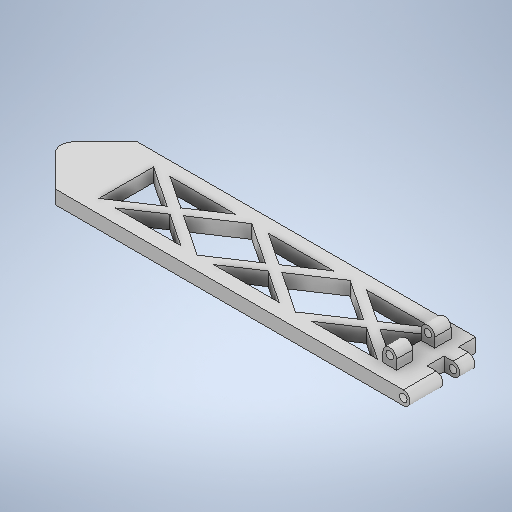
# Autodesk Inventor part: scrambler_spider_beam
Saved by Autodesk Inventor 2025.2 (Build 292293000, 293)
## iProperties
Created: 2025-10-10
Part Number: scrambler_spider_beam
Material: Generic
Document SubType Name: Modeling
Designer: pascu
Density: 1 g/cm^3
Appearance: Default
Author: pascu
Autodesk Inventor part; units mm, degrees
ref_plane "YZ Plane" through (0, 0, 0) normal (1, 0, 0) x (0, 1, 0)
ref_plane "XZ Plane" through (0, 0, 0) normal (0, 1, 0) x (-1, 0, 0)
ref_plane "XY Plane" through (0, 0, 0) normal (0, 0, 1) x (1, 0, 0)
sketch "Sketch1" plane through (0, 0, 0) normal (0, 1, 0) x (-1, 0, 0)
  line L0 (0, 0) -> (-82.55, 0)
  line L1 (-82.55, 0) -> (-82.55, -19.05)
  line L2 (-82.55, -19.05) -> (0, -19.05)
  line L3 (0, -19.05) -> (0, 0)
  dimension "d0" = 82.55
  dimension "d1" = 19.05
  constraints: 8 end point, 2 parallel, 1 horizontal, 1 perpendicular
  measures "d0" distance of L2.end L1.end
  measures "d1" distance of L1.end L0.end
extrude "Extrusion1" add sketch "Sketch1" along normal blind 3.175
sketch "Sketch2" plane through (0, 3.175, 0) normal (0, 1, 0) x (1, 0, 0)
  line L0 (6.985, 15.875) -> (75.565, 15.875) construction
  line L1 (75.565, 15.875) -> (75.565, 3.175) construction
  line L2 (75.565, 3.175) -> (6.985, 3.175) construction
  line L3 (6.985, 3.175) -> (6.985, 15.875) construction
  line L4 (0, 0) -> (82.55, 0) construction
  line L5 (82.55, 0) -> (82.55, 19.05) construction
  line L6 (6.985, 3.175) -> (29.845, 3.175) construction
  line L7 (6.985, 15.875) -> (10.795, 15.875) construction
  line L8 (10.795, 15.875) -> (18.415, 10.795)
  line L9 (6.985, 15.875) -> (16.51, 9.525)
  line L10 (6.985, 9.525) -> (11.4454, 9.525) construction
  line L11 (10.795, 3.175) -> (18.415, 8.255)
  line L12 (6.985, 3.175) -> (16.51, 9.525)
  line L13 (6.985, 15.875) -> (6.985, 3.175)
  line L14 (10.795, 3.175) -> (26.035, 3.175)
  line L15 (10.795, 15.875) -> (26.035, 15.875)
  line L16 (18.415, 10.795) -> (26.035, 15.875)
  line L17 (20.32, 9.525) -> (29.845, 15.875)
  line L18 (18.415, 8.255) -> (26.035, 3.175)
  line L19 (20.32, 9.525) -> (29.845, 3.175)
  line L20 (43.18, 9.525) -> (52.705, 3.175)
  line L21 (41.275, 8.255) -> (48.895, 3.175)
  line L22 (43.18, 9.525) -> (52.705, 15.875)
  line L23 (41.275, 10.795) -> (48.895, 15.875)
  line L24 (33.655, 15.875) -> (48.895, 15.875)
  line L25 (33.655, 3.175) -> (48.895, 3.175)
  line L26 (33.655, 3.175) -> (41.275, 8.255)
  line L27 (29.845, 3.175) -> (39.37, 9.525)
  line L28 (29.845, 15.875) -> (39.37, 9.525)
  line L29 (33.655, 15.875) -> (41.275, 10.795)
  line L30 (66.04, 9.525) -> (75.565, 3.175)
  line L31 (64.135, 8.255) -> (71.755, 3.175)
  line L32 (66.04, 9.525) -> (75.565, 15.875)
  line L33 (64.135, 10.795) -> (71.755, 15.875)
  line L34 (56.515, 15.875) -> (71.755, 15.875)
  line L35 (56.515, 3.175) -> (71.755, 3.175)
  line L36 (56.515, 3.175) -> (64.135, 8.255)
  line L37 (52.705, 3.175) -> (62.23, 9.525)
  line L38 (52.705, 15.875) -> (62.23, 9.525)
  line L39 (56.515, 15.875) -> (64.135, 10.795)
  line L40 (75.565, 15.875) -> (75.565, 3.175)
  point P0 (29.845, 3.175)
  dimension "d4" = 68.58
  dimension "d5" = 12.7
  dimension "d6" = 3.175
  dimension "d7" = 6.985
  dimension "d8" = 22.86
  dimension "d9" = 3.81
  dimension "d12" = 22.86
  constraints: 78 end point, 8 point on line, 6 parallel, 3 horizontal, 3 symmetric about line, 2 collinear, 1 midpoint, 1 perpendicular, 1 vertical, 44 other
  measures "d4" distance between parallel lines of L3 L1
  measures "d5" distance of L0.end L1.end
  measures "d6" distance between parallel lines of L4 L2
  measures "d7" distance between parallel lines of L5 L1
  measures "d8" distance of L2.end L6.end
  measures "d9" distance of L0.start L7.end
  measures "d12" distance of L17.start L20.start
extrude "Extrusion2" cut sketch "Sketch2" against normal blind 3.81
fillet "Fillet2" radius 1.5875 2 edges at (82.55, 0, -9.525) (82.55, 3.175, -9.525)
ref_plane "Work Plane1" through (1.5875, 1.5875, 0) normal (0, 0, 1) x (1, 0, 0)
sketch "Sketch3" plane through (1.5875, 1.5875, 0) normal (0, 0, 1) x (1, 0, 0)
  arc A0 (79.375, -1.5875) -> (79.375, 1.5875) centre (79.375, 0) ccw projected
  point P0 (-1.5875, -1.5875)
  constraints: 1 coincident
hole "Hole1" at (80.9625, 1.5875, 0) direction (0, 0, -1) diameter 1.778 end through all
sketch "Sketch4" plane through (0, 3.175, 0) normal (0, 1, 0) x (1, 0, 0)
  line L0 (82.55, 0) -> (82.55, 19.05) projected
  line L1 (82.55, 19.05) -> (78.74, 19.05)
  line L2 (78.74, 19.05) -> (78.74, 15.113)
  line L3 (78.74, 15.113) -> (82.55, 15.113)
  line L4 (82.55, 15.113) -> (82.55, 19.05)
  line L5 (82.55, 15.113) -> (82.55, 11.557)
  line L6 (82.55, 11.557) -> (78.8818, 11.557)
  line L7 (78.8818, 11.557) -> (78.8818, 7.62)
  line L8 (78.8818, 7.62) -> (82.55, 7.62)
  line L9 (82.55, 7.62) -> (82.55, 11.557)
  point P0 (0, 0)
  dimension "d28" = 3.81
  dimension "d29" = 3.937
  dimension "d30" = 3.556
  dimension "d31" = 3.937
  constraints: 18 end point, 4 perpendicular, 3 point on line, 2 parallel, 1 collinear, 1 horizontal
  measures "d28" distance of L3.end L2.end
  measures "d29" distance of L2.end L1.end
  measures "d30" distance of L3.end L5.end
  measures "d31" distance of L6.end L7.end
extrude "Extrusion3" cut sketch "Sketch4" against normal blind 3.175
sketch "Sketch5" plane through (0, 0, 0) normal (0, -1, 0) x (1, 0, 0)
  circle A0 centre (-9.525, -9.525) radius 15.875 projected
  line L0 (0, 0) -> (-7.2799, -7.2799)
  line L1 (-7.2799, -11.7701) -> (0, -19.05)
  line L2 (0, -19.05) -> (0, 0) projected
  line L3 (0, -19.05) -> (0, 0) projected
  line L4 (0, -19.05) -> (0, 0)
  arc A1 (-7.2799, -7.2799) -> (-7.2799, -11.7701) centre (-5.0349, -9.525) ccw
  dimension "d34" = 3.175
  constraints: 6 end point, 2 point on circle, 2 point on line, 2 tangent, 1 centre point, 1 collinear, 1 perpendicular
  measures "d34" radius of A1
extrude "Extrusion4" add sketch "Sketch5" against normal blind 3.175 contours L2 L1 A1 L0
sketch "Sketch6" plane through (0, 3.175, 0) normal (0, 1, 0) x (1, 0, 0)
  line L0 (75.565, 15.875) -> (75.565, 3.175) projected
  line L1 (75.565, 9.525) -> (75.565, 6.985)
  line L2 (75.565, 3.175) -> (75.565, 15.875)
  line L3 (66.04, 9.525) -> (75.565, 15.875) projected
  line L4 (75.565, 15.875) -> (73.025, 15.875) construction
  line L5 (75.565, 3.175) -> (66.04, 9.525) projected
  line L6 (75.565, 3.175) -> (73.025, 4.8683)
  line L7 (73.025, 14.1817) -> (73.025, 4.8683)
  line L8 (73.025, 14.1817) -> (75.565, 15.875)
  point P0 (0, 0)
  dimension "d38" = 2.54
  constraints: 12 end point, 4 point on line, 2 vertical, 1 collinear, 1 midpoint, 1 perpendicular
  measures "d38" distance of L0.start L4.end
extrude "Extrusion5" add sketch "Sketch6" against normal blind 3.175 contours L0 L5 L7 L3
sketch "Sketch7" plane through (0, 3.175, 0) normal (0, 1, 0) x (1, 0, 0)
  line L0 (73.025, 4.8683) -> (73.025, 14.1817) projected
  line L1 (73.025, 9.525) -> (73.025, 6.985)
  line L2 (73.025, 6.985) -> (76.2, 6.985)
  line L3 (76.2, 6.985) -> (76.2, 3.175)
  line L4 (76.2, 3.175) -> (73.025, 3.175)
  line L5 (73.025, 3.175) -> (73.025, 6.985)
  line L6 (73.025, 9.525) -> (73.025, 12.065)
  line L7 (73.025, 12.065) -> (76.2, 12.065)
  line L8 (76.2, 12.065) -> (76.2, 15.875)
  line L9 (76.2, 15.875) -> (73.025, 15.875)
  line L10 (73.025, 15.875) -> (73.025, 12.065)
  point P0 (0, 0)
  dimension "d41" = 2.54
  dimension "d42" = 3.175
  dimension "d43" = 3.81
  dimension "d44" = 2.54
  dimension "d45" = 3.175
  dimension "d46" = 3.81
  constraints: 20 end point, 5 perpendicular, 3 point on line, 2 collinear, 1 midpoint, 1 vertical
  measures "d41" distance of L1.start L1.end
  measures "d42" distance of L1.end L2.end
  measures "d43" distance of L2.end L3.end
  measures "d44" distance of L1.start L6.end
  measures "d45" distance of L6.end L7.end
  measures "d46" distance of L7.end L8.end
extrude "Extrusion6" add sketch "Sketch7" along normal blind 3.81
fillet "Fillet3" radius 1.5875 4 edges at (73.025, 6.985, -13.97) (76.2, 6.985, -13.97) (73.025, 6.985, -5.08) (76.2, 6.985, -5.08)
sketch "Sketch8" plane through (76.2, 3.175, -15.875) normal (0, 0, -1) x (-1, 0, 0)
  arc A0 (3.175, 2.2225) -> (0, 2.2225) centre (1.5875, 2.2225) ccw projected
  circle A1 centre (1.5875, 2.2225) radius 0.889
  point P0 (76.2, -3.175)
  dimension "d50" = 1.778
  constraints: 1 centre point, 1 coincident
  measures "d50" diameter of A1
extrude "Extrusion7" cut sketch "Sketch8" against normal through all
body "Solid1"
